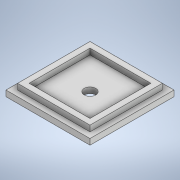
# Autodesk Inventor part: waterBallonHolderCapv2
Saved by Autodesk Inventor 2020.5 (Build 245400000, 400)
## iProperties
Created: 2022-09-15
Part Number: waterBallonHolderCapv2
Material: Generic
Document SubType Name: Modeling
Designer: kouda
Density: 1 g/cm^3
Appearance: Default
Author: kouda
Autodesk Inventor part; units mm, degrees
ref_plane "YZ Plane" through (0, 0, 0) normal (1, 0, 0) x (0, 1, 0)
ref_plane "XZ Plane" through (0, 0, 0) normal (0, 1, 0) x (-1, 0, 0)
ref_plane "XY Plane" through (0, 0, 0) normal (0, 0, 1) x (1, 0, 0)
sketch "Sketch3" plane through (0, 0, 0) normal (0, 1, 0) x (-1, 0, 0)
  line L0 (0, 0) -> (29, 0)
  line L1 (29, 0) -> (29, -29)
  line L2 (29, -29) -> (0, -29)
  line L3 (0, -29) -> (0, 0)
  dimension "d8" = 29
  dimension "d9" = 29
  constraints: 8 end point, 2 parallel, 1 horizontal, 1 perpendicular
  measures "d8" distance of L1.end L2.end
  measures "d9" distance of L0.end L1.end
extrude "Extrusion3" add sketch "Sketch3" along normal blind 2
sketch "Sketch4" plane through (0, 2, 0) normal (0, 1, 0) x (1, 0, 0)
  line L0 (-29, 29) -> (-29, 0) projected
  line L1 (-29, 0) -> (0, 0) projected
  line L2 (0, 0) -> (0, 29) projected
  line L3 (0, 29) -> (-29, 29) projected
  line L4 (-27, 2) -> (-27, 27)
  line L5 (-27, 27) -> (-2, 27)
  line L6 (-2, 27) -> (-2, 2)
  line L7 (-2, 2) -> (-27, 2)
  line L8 (-25, 25) -> (-25, 4)
  line L9 (-25, 4) -> (-4, 4)
  line L10 (-4, 4) -> (-4, 25)
  line L11 (-4, 25) -> (-25, 25)
  dimension "d12" = 2
  dimension "d13" = 2
  constraints: 16 end point, 6 other
  measures "d12" distance between parallel lines of L0 L4
  measures "d13" distance between parallel lines of L4 L8
extrude "Extrusion4" add sketch "Sketch4" along normal blind 2 contours L4 L5 L6 L7
sketch "Sketch5" plane through (0, 0, 0) normal (0, -1, 0) x (1, 0, 0)
  line L0 (-4, -4) -> (-4, -25) projected
  line L1 (-4, -25) -> (-25, -25) projected
  line L2 (-25, -25) -> (-25, -4) projected
  line L3 (-25, -4) -> (-4, -4) projected
  line L4 (-4, -4) -> (-14, -4)
  line L5 (-14, -4) -> (-14, -14)
  line L6 (-14, -14) -> (-4, -14)
  line L7 (-4, -14) -> (-4, -4)
  point P0 (0, 0)
  dimension "d16" = 10
  dimension "d17" = 10
  constraints: 8 end point, 2 parallel, 1 coincident, 1 horizontal, 1 perpendicular
  measures "d16" distance of L6.end L5.end
  measures "d17" distance of L5.end L4.end
hole "Hole1" at (-14, 0, -14) direction (0, 1, 0) diameter 4 end through all
body "Solid2"
